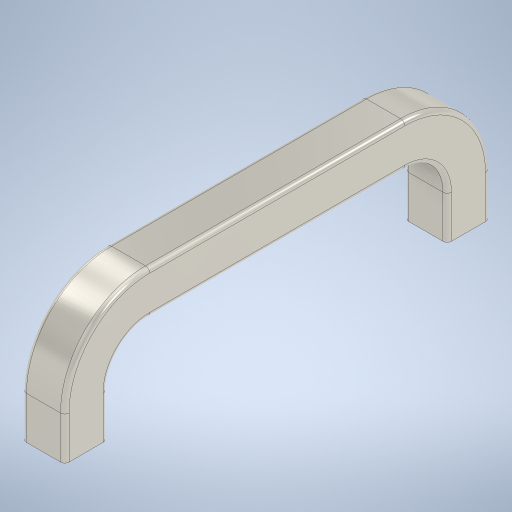
# Autodesk Inventor part: Handle_Part
Saved by Autodesk Inventor 2024 (Build 280153000, 153)
## iProperties
Created: 2024-05-20
Part Number: Handle_Part
Material: Generic
Document SubType Name: Modeling
Designer: ASUS
Density: 1 g/cm^3
Appearance: Default
Author: ASUS
Autodesk Inventor part; units mm, degrees
ref_plane "YZ Plane" through (0, 0, 0) normal (1, 0, 0) x (0, 1, 0)
ref_plane "XZ Plane" through (0, 0, 0) normal (0, 1, 0) x (-1, 0, 0)
ref_plane "XY Plane" through (0, 0, 0) normal (0, 0, 1) x (1, 0, 0)
sketch "Sketch1" plane through (0, 0, 0) normal (0, 1, 0) x (-1, 0, 0)
  line L0 (10, 100) -> (-10, 100)
  line L1 (-10, 100) -> (-10, 80)
  line L2 (-10, 80) -> (10, 80)
  line L3 (10, 80) -> (10, 100)
  line L4 (10, 100) -> (-10, 80) construction
  line L5 (-10, 100) -> (10, 80) construction
  line L6 (10, -80) -> (-10, -80)
  line L7 (-10, -80) -> (-10, -100)
  line L8 (-10, -100) -> (10, -100)
  line L9 (10, -100) -> (10, -80)
  line L10 (10, -80) -> (-10, -100) construction
  line L11 (-10, -80) -> (10, -100) construction
  point P0 (0, 0)
  point P1 (0, 90)
  point P2 (0, -90)
  dimension "d0" = 20
  dimension "d1" = 20
  dimension "d2" = 20
  dimension "d3" = 20
  dimension "d4" = 80
  dimension "d5" = 80
  dimension "d6" = 0
  constraints: 24 end point, 4 midpoint, 4 parallel, 2 horizontal, 2 perpendicular, 1 point on line
  measures "d0" distance of L7.end L8.end
  measures "d1" distance of L8.end L6.start
  measures "d2" distance of L1.end L2.end
  measures "d3" distance of L2.end L0.start
  measures "d4" distance from line of L6 point (0, 0)
  measures "d5" distance from line of point (0, 0) L2
  measures "d6" horizontal distance of point (0, 0) point (0, 90)
extrude "Extrusion1" add sketch "Sketch1" along normal blind 40
sketch "Sketch2" plane through (-10, 0, 100) normal (0, 0, 1) x (1, 0, 0)
  line L0 (0, 0) -> (0, 40) projected
  line L1 (0, 40) -> (20, 40)
  line L2 (20, 40) -> (20, 60)
  line L3 (20, 60) -> (0, 60)
  line L4 (0, 60) -> (0, 40)
  point P0 (10, 0)
  dimension "d9" = 20
  dimension "d10" = 20
  constraints: 8 end point, 2 parallel, 1 horizontal, 1 perpendicular
  measures "d9" distance of L2.end L3.end
  measures "d10" distance of L1.end L2.end
extrude "Extrusion2" add sketch "Sketch2" against normal blind 200
fillet "Fillet1" radius 20 2 edges at (0, 40, -80) (0, 40, 80)
fillet "Fillet2" radius 40 2 edges at (0, 60, 100) (0, 60, -100)
fillet "Fillet3" radius 2 10 edges at (10, 40, 0) (10, 34.1421, -74.1421) (10, 10, -80) (10, 34.1421, 74.1421) (10, 10, 80) (10, 10, -100) (10, 48.2843, -88.2843) (10, 60, 0) (10, 48.2843, 88.2843) (10, 10, 100)
fillet "Fillet4" radius 2 10 edges at (-10, 10, -80) (-10, 34.1421, -74.1421) (-10, 40, 0) (-10, 34.1421, 74.1421) (-10, 10, 80) (-10, 48.2843, 88.2843) (-10, 10, 100) (-10, 60, 0) (-10, 48.2843, -88.2843) (-10, 10, -100)
shell "Shell1" thickness 2 removed faces 2 at (-2.6667, 0, -93.3333) at (2.6667, 0, 93.3333)
sketch "Sketch3" plane through (0, 0, 0) normal (0, -1, 0) x (1, 0, 0)
  line L0 (-8, -82) -> (8, -82) projected
  line L1 (-8, -98) -> (8, -98)
  line L2 (8, -98) -> (8, -82)
  line L3 (8, -82) -> (-8, -82)
  line L4 (-8, -82) -> (-8, -98)
  line L5 (8, -98) -> (-8, -98) projected
  line L6 (-8, -98) -> (-8, -82) projected
  point P0 (0, 0)
  constraints: 8 end point, 2 collinear, 2 parallel, 1 horizontal, 1 perpendicular
extrude "Extrusion3" add sketch "Sketch3" against normal blind 10
mirror "Mirror1" about plane through (0, 0, 0) normal (0, 0, 1) of "Extrusion3"
sketch "Sketch4" plane through (0, 0, 0) normal (0, -1, 0) x (1, 0, 0)
  circle A0 centre (0, 90) radius 2.5
  line L0 (-8, 100) -> (8, 100) projected
  line L1 (-10, 82) -> (-10, 98) projected
  point P0 (0, 0)
  dimension "d20" = 5
  dimension "d21" = 10
  dimension "d22" = 10
  constraints: 1 centre point
  measures "d20" diameter of A0
  measures "d21" distance from line of L0 A0.centre
  measures "d22" distance from line of L1 A0.centre
extrude "Extrusion4" cut sketch "Sketch4" against normal blind 5
thread "Thread1" size "M5x0.8" class "6H" standard "ISO Metric profile" full length
mirror "Mirror2" about plane through (0, 0, 0) normal (0, 0, 1) of "Extrusion4"
body "Solid1"
